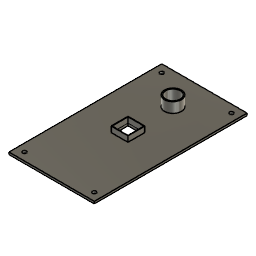
FINAL PROJECT V1-cover (Autodesk Fusion 360 design; units mm, degrees)
part number: 2026-05-25-17-51-36-576
Autodesk Fusion 360 part; units mm, degrees
sketch "Sketch1" plane through (0, 0, 0) normal (0, 0, 1) x (1, 0, 0)
  line L0 (38, 68) -> (-38, 68)
  line L1 (-38, 68) -> (-38, -68)
  line L2 (-38, -68) -> (38, -68)
  line L3 (38, -68) -> (38, 68)
  line L4 (38, 68) -> (-38, -68) construction
  line L5 (-38, 68) -> (38, -68) construction
  line L6 (7.1, 7.1) -> (-7.1, 7.1)
  line L7 (-7.1, 7.1) -> (-7.1, -7.1)
  line L8 (-7.1, -7.1) -> (7.1, -7.1)
  line L9 (7.1, -7.1) -> (7.1, 7.1)
  line L10 (7.1, 7.1) -> (-7.1, -7.1) construction
  line L11 (-7.1, 7.1) -> (7.1, -7.1) construction
  circle A0 centre (0, 40) radius 6.5
  circle A1 centre (0, 40) radius 7.5
  line L12 (-38, 68) -> (-31, 68)
  line L13 (-31, 68) -> (-31, 61)
  line L14 (-31, 61) -> (-38, 61)
  line L15 (-38, 61) -> (-38, 68)
  circle A2 centre (-31, 61) radius 1.7
  line L16 (38, 68) -> (31, 68)
  line L17 (31, 68) -> (31, 61)
  line L18 (31, 61) -> (38, 61)
  line L19 (38, 61) -> (38, 68)
  circle A3 centre (31, 61) radius 1.7
  circle A4 centre (-31, -61) radius 1.7
  circle A5 centre (31, -61) radius 1.7
  line L20 (7.5, 7.5) -> (-7.5, 7.5)
  line L21 (-7.5, 7.5) -> (-7.5, -7.5)
  line L22 (-7.5, -7.5) -> (7.5, -7.5)
  line L23 (7.5, -7.5) -> (7.5, 7.5)
  line L24 (7.5, 7.5) -> (-7.5, -7.5) construction
  line L25 (-7.5, 7.5) -> (7.5, -7.5) construction
  dimension "d1" = 76
  dimension "d2" = 136
  dimension "d3" = 14.2
  dimension "d4" = 14.2
  dimension "d5" = 13
  dimension "d6" = 1
  dimension "d7" = 7
  dimension "d8" = 7
  dimension "d9" = 3.4
  dimension "d10" = 7
  dimension "d11" = 7
  dimension "d14" = 62
  dimension "d15" = -122
  dimension "d16" = 15
  dimension "d17" = 15
  constraint horizontal L0
  constraint perpendicular L0 L1
  constraint parallel L0 L2
  constraint parallel L1 L3
  constraint coincident L4 origin
  constraint coincident L5 origin
  constraint horizontal L6
  constraint perpendicular L6 L7
  constraint parallel L6 L8
  constraint parallel L7 L9
  constraint coincident L10 origin
  constraint coincident L11 origin
  constraint horizontal L12
  constraint vertical L13
  constraint horizontal L14
  constraint vertical L15
  constraint coincident L13.end L14.start
  constraint horizontal L16
  constraint vertical L17
  constraint horizontal L18
  constraint vertical L19
  constraint horizontal L20
  constraint perpendicular L20 L21
  constraint parallel L20 L22
  constraint parallel L21 L23
  constraint coincident L24 origin
  constraint coincident L25 origin
  measures "d1" distance of L1.end L2.end
  measures "d2" distance of L0.end L1.end
  measures "d3" distance of L7.end L8.end
  measures "d4" distance of L6.end L7.end
  measures "d5" diameter of A0
  measures "d7" distance of L0.end L12.end
  measures "d8" distance of L0.end L14.end
  measures "d9" diameter of A2
  measures "d10" distance of L0.start L16.end
  measures "d11" distance of L0.start L18.end
  measures "d16" distance of L21.end L22.end
  measures "d17" distance of L20.end L21.end
extrude "Extrude1" add sketch "Sketch1" along normal blind 2 contours L0 L3 L16 L17 L18 L19 A3 | L0 L1 L2 L3 L13 L14 A2 L17 L18 A3 | L0 L1 L12 L13 L14 L15 A2
extrude "Extrude2" add sketch "Sketch1" along normal blind 11 contours A1
extrude "Extrude3" add sketch "Sketch1" along normal blind 7 contours L20 L21 L22 L23
